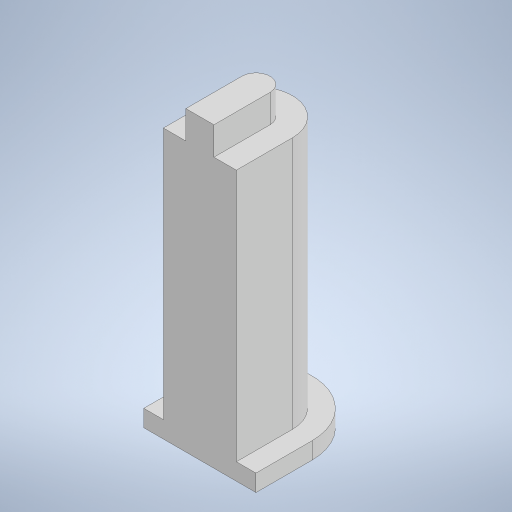
# Autodesk Inventor part: Stand
Saved by Autodesk Inventor 2024.1 (Build 281209000, 209)
## iProperties
Created: 2023-12-30
Part Number: Stand
Material: Generic
Document SubType Name: Modeling
Designer: ryanm
Density: 1 g/cm^3
Appearance: Default
Author: ryanm
Autodesk Inventor part; units mm, degrees
ref_plane "YZ Plane" through (0, 0, 0) normal (1, 0, 0) x (0, 1, 0)
ref_plane "XZ Plane" through (0, 0, 0) normal (0, 1, 0) x (-1, 0, 0)
ref_plane "XY Plane" through (0, 0, 0) normal (0, 0, 1) x (1, 0, 0)
sketch "Sketch1" plane through (0, 0, 0) normal (0, 1, 0) x (-1, 0, 0)
  arc A0 (-10, 0) -> (10, 0) centre (0, 0) ccw
  line L0 (10, 0) -> (10, 10)
  line L1 (10, 10) -> (-10, 10)
  line L2 (-10, 10) -> (-10, 0)
  dimension "d0" = 20
  dimension "d9" = 10
  dimension "d10" = 10
  dimension "d11" = 20
  constraints: 6 end point, 2 perpendicular, 2 point on circle, 1 centre point, 1 coincident, 1 vertical
  measures "d0" diameter of A0
  measures "d9" distance of L0.start L0.end
  measures "d10" distance of L2.end L1.end
  measures "d11" distance of L0.end L1.end
extrude "Extrusion1" add sketch "Sketch1" along normal blind 3
sketch "Sketch2" plane through (0, 3, 0) normal (0, 1, 0) x (-1, 0, 0)
  arc A0 (-6.5, 0) -> (6.5, 0) centre (0, 0) ccw
  line L0 (6.5, 0) -> (6.5, 10)
  line L1 (10, 10) -> (-10, 10) projected
  line L2 (-6.5, 10) -> (-6.5, 0)
  dimension "d3" = 13
  constraints: 4 end point, 2 point on circle, 2 point on line, 2 tangent, 1 centre point, 1 coincident, 1 parallel, 1 vertical
  measures "d3" diameter of A0
extrude "Extrusion2" add sketch "Sketch2" along normal blind 45
sketch "Sketch3" plane through (0, 48, 0) normal (0, 1, 0) x (-1, 0, 0)
  arc A0 (-2.5, 0) -> (2.5, 0) centre (0, 0) ccw
  line L0 (2.5, 0) -> (2.5, 10)
  line L1 (-2.5, 0) -> (-2.5, 10)
  line L2 (6.5, 0) -> (6.5, 10) projected
  line L3 (6.5, 10) -> (-6.5, 10) projected
  line L4 (-6.5, 10) -> (-6.5, 0) projected
  arc A1 (-6.5, 0) -> (6.5, 0) centre (0, 0) ccw projected
  point P0 (2.5, 10)
  dimension "d6" = 5
  dimension "d12" = 5
  constraints: 4 end point, 2 horizontal alignment, 2 point on circle, 2 vertical, 1 centre point, 1 coincident, 1 tangent
  measures "d6" diameter of A0
  measures "d12" distance between parallel lines of L1 L0
extrude "Extrusion3" add sketch "Sketch3" along normal blind 5 contours L1 L3 L0 A0
equation "\"d12\" = d6"
body "Solid1"
